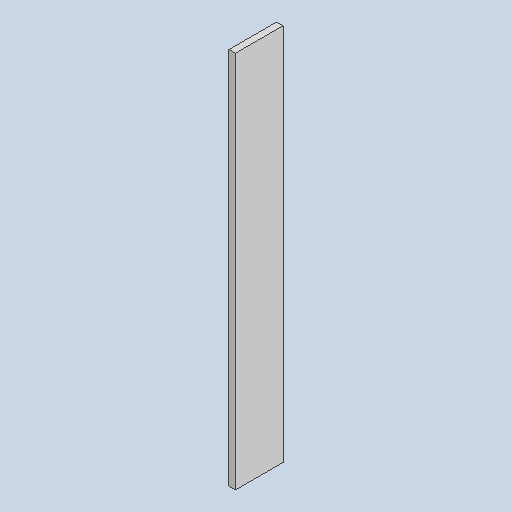
# Autodesk Inventor part: ДМФ 01 58 Фиксатор расстояния кассет
Saved by Autodesk Inventor 2024.2 (Build 282272000, 272)
## iProperties
Created: 2024-05-05
Part Number: ДМФ 01 58 Фиксатор расстояния кассет
Material: Generic
Document SubType Name: Modeling
Designer: pokla
Density: 1 g/cm^3
Appearance: Default
Author: pokla
Autodesk Inventor part; units mm, degrees
ref_plane "YZ Plane" through (0, 0, 0) normal (1, 0, 0) x (0, 1, 0)
ref_plane "XZ Plane" through (0, 0, 0) normal (0, 1, 0) x (-1, 0, 0)
ref_plane "XY Plane" through (0, 0, 0) normal (0, 0, 1) x (1, 0, 0)
sketch "Sketch1" plane through (0, 0, 0) normal (0, 0, 1) x (1, 0, 0)
  line L0 (0, 277.6336) -> (196.3166, 196.3166) construction
  line L1 (196.3166, 196.3166) -> (277.6336, 0) construction
  line L2 (277.6336, 0) -> (196.3166, -196.3166) construction
  line L3 (196.3166, -196.3166) -> (0, -277.6336) construction
  line L4 (0, -277.6336) -> (-196.3166, -196.3166) construction
  line L5 (-196.3166, -196.3166) -> (-277.6336, 0) construction
  line L6 (-277.6336, 0) -> (-196.3166, 196.3166) construction
  line L7 (-196.3166, 196.3166) -> (0, 277.6336) construction
  line L8 (-196.3166, 196.3166) -> (0, 277.6336) construction
  line L9 (-461.2666, 773.8898) -> (-221.0579, 873.3874) construction
  line L10 (-98.1583, 236.9751) -> (-341.1623, 823.6386) construction
  line L11 (-221.0579, 873.3874) -> (0, 873.3874) construction
  line L12 (0, 873.3874) -> (0, 277.6336) construction
  line L13 (-461.2666, 773.8898) -> (-617.5782, 617.5782) construction
  line L14 (-617.5782, 617.5782) -> (-196.3166, 196.3166) construction
  line L15 (-5, 868.3874) -> (-220.0634, 868.3874) construction
  line L16 (-220.0634, 868.3874) -> (-458.4343, 769.651) construction
  line L17 (-458.4343, 769.651) -> (-610.5071, 617.5782) construction
  line L18 (-610.5071, 617.5782) -> (-195.1434, 202.2145) construction
  line L19 (-195.1434, 202.2145) -> (-5, 280.9745) construction
  line L20 (-5, 280.9745) -> (-5, 868.3874)
  line L21 (-5, 868.3874) -> (-5, 280.9745) construction
  line L22 (5, 868.3874) -> (5, 280.9745)
  line L23 (-5, 280.9745) -> (5, 280.9745)
  line L24 (-5, 868.3874) -> (5, 868.3874)
  point P0 (0, 0)
  point P1 (0, 0)
  point P2 (0, 0)
  dimension "d0" = 513
  dimension "d1" = 260
  dimension "d2" = 635
  dimension "d6" = 5
  constraints: 50 end point, 3 horizontal, 2 coincident, 2 midpoint, 2 parallel, 2 vertical, 1 collinear, 1 horizontal alignment, 1 perpendicular, 1 symmetric about line, 1 vertical alignment, 23 other
  measures "d0" distance between parallel lines of L5 L1
  measures "d1" distance of L9.start L11.start
  measures "d2" distance of L10.end L10.start
  measures "d6" distance between parallel lines of L11 L15
extrude "Extrusion1" add sketch "Sketch1" along normal mid plane 74
equation "\"d0\" = Барабан_габарит_по_кассетам"
equation "\"d1\" = Кассета_длина_грани"
equation "\"d2\" = Кассета_высота"
equation "\"Барабан_габарит_по_кассетам\" = 513"
equation "\"Кассета_длина_грани\" = 260"
equation "\"Кассета_высота\" = 635"
body "Solid1"
